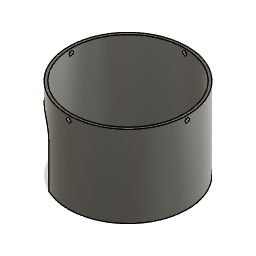
CylinderSupport v2 (Autodesk Fusion 360 design; units mm, degrees)
Autodesk Fusion 360 part; units mm, degrees
sketch "Sketch1" plane through (0, 0, 0) normal (0, 1, 0) x (1, 0, 0)
  circle A0 centre (0, 0) radius 65
  circle A1 centre (0, 0) radius 68
  dimension "d1" = 130
  dimension "d2" = 3
  constraint coincident A0.centre A1.centre
  measures "d1" diameter of A0
extrude "Extrude1" add sketch "Sketch1" along normal blind 93.5
sketch "Sketch2" plane through (0, 0, 0) normal (0, 0, 1) x (1, 0, 0)
  line L0 (-22.5, 0) -> (22.5, 0)
  line L1 (22.5, 0) -> (22.5, 50)
  line L2 (22.5, 50) -> (-22.5, 50) construction
  line L3 (-22.5, 50) -> (-22.5, 0)
  circle A0 centre (0, 50) radius 22.5
  dimension "d5" = 45
  dimension "d6" = 50
  constraint horizontal L0
  constraint vertical L1
  constraint horizontal L2
  constraint vertical L3
  constraint coincident L1.end A0
  constraint tangent L1 A0
  constraint coincident L2.end A0
  constraint midpoint origin L0
  measures "d5" distance of L0.start L0.end
  measures "d6" distance of L0.start L2.end
extrude "Extrude2" cut sketch "Sketch2" along normal blind 110
sketch "Sketch3" plane through (0, 0, 0) normal (1, 0, 0) x (0, 0, -1)
  circle A0 centre (0, 88.5) radius 2.5
  dimension "d9" = 88.5
  dimension "d10" = 5
  measures "d9" distance of origin A0.centre
  measures "d10" diameter of A0
move_body "Move1" bodies 1 to x (0.707107, 0, 0.707107) y (0, 1, 0) z (-0.707107, 0, 0.707107) at (0, 0, 0)
extrude "Extrude3" cut sketch "Sketch3" along normal mid plane 270
sketch "Sketch4" plane through (0, 0, 0) normal (0, 0, 1) x (1, 0, 0)
  circle A0 centre (0, 88.5) radius 2.5
  dimension "d13" = 88.5
  dimension "d14" = 5
  measures "d13" distance of A0.centre origin
  measures "d14" diameter of A0
extrude "Extrude4" cut sketch "Sketch4" along normal mid plane 170
